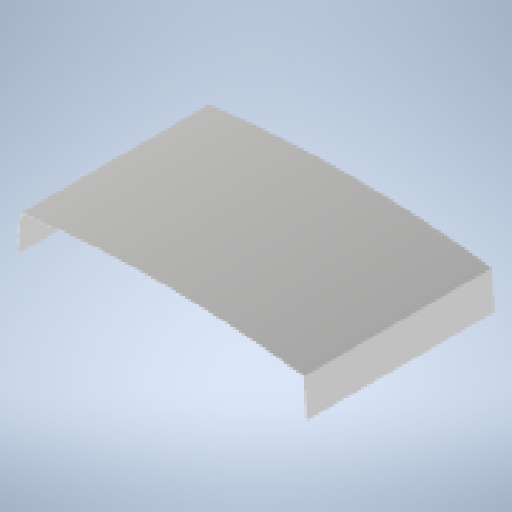
# Autodesk Inventor part: МОО 010 лист спина 1
Saved by Autodesk Inventor 2024.2 (Build 282272000, 272)
## iProperties
Created: 2024-04-18
Part Number: МОО 010 лист спина 1
Material: Stainless Steel AISI 304
Document SubType Name: Sheet Metal
Designer: admin
Density: 8 g/cm^3
Flat Pattern Width: 100 cm
Flat Pattern Length: 190.053 cm
Flat Pattern Area: 19005.3 cm^2
Sheet Metal Rule: Default_mm
Sheet Metal Width: 1000,000 mm
Sheet Metal Length: 1900,535 mm
Sheet Metal Area: 1900534,780 mm^2
Appearance: Default
Mass: 48037.2 g
Surface Area: 40211.1 cm^2
Volume: 6004.65 cm^3
Stock Number: МОО 010 лист спина 1
Author: admin
Autodesk Inventor part; units mm, degrees
ref_plane "YZ Plane" through (0, 0, 0) normal (1, 0, 0) x (0, 1, 0)
ref_plane "XZ Plane" through (0, 0, 0) normal (0, 1, 0) x (-1, 0, 0)
ref_plane "XY Plane" through (0, 0, 0) normal (0, 0, 1) x (1, 0, 0)
sketch "Sketch1" plane through (0, 0, 0) normal (0, 0, 1) x (1, 0, 0)
  line L0 (-800, -50) -> (800, -50) construction
  line L1 (800, -50) -> (800, 0) construction
  line L2 (800, 0) -> (-800, 0) construction
  line L3 (-800, 0) -> (-800, -50) construction
  arc A0 (750, -50) -> (-750, -50) centre (0, -5650) ccw
  arc A1 (-750, -50) -> (-752.5925, -52.7381) centre (-749.6018, -52.9735) ccw
  line L4 (-752.5925, -52.7381) -> (-767.6567, -244.1462)
  arc A2 (752.5925, -52.7381) -> (750, -50) centre (749.6018, -52.9735) ccw
  line L5 (752.5925, -52.7381) -> (767.6567, -244.1462)
  line L6 (0, 0) -> (0, -50) construction
  dimension "d0" = 1600
  dimension "d1" = 50
  dimension "d2" = 50
  dimension "d14" = 3
  dimension "d15" = 192
  dimension "d16" = 94.5
  measures "d0" distance of L2.end L1.end
  measures "d1" distance of L1.end L0.end
  measures "d2" distance of L0.start A0.end
  measures "d14" radius of A1
  measures "d15" distance of L4.start L4.end
  measures "d16" angle of L4 L0
contour flange "Contour Flange1" sketch "Sketch1" thickness 3 bend radius 3 width 1000 along (0, 0, 1) mid plane no both sides no wall seen from (760.1246, -148.4421, 0) lies toward (0.9969173, 0.0784591, 0) curves L5 A2 A0 A1 L4
bend "Bend1"
corner "Corner1"
equation "\"d2\" = d1"
equation "\"d14\" = BendRadius"
equation "\"d3\" = Thickness"
equation "\"d4\" = BendReliefWidth"
equation "\"d5\" = BendReliefDepth"
equation "\"d6\" = MinimumRemnant"
equation "\"d7\" = TransitionRadius"
equation "\"d9\" = BendRadius"
equation "\"d11\" = CornerReliefSize"
equation "\"d12\" = GapSize"
equation "\"d13\" = JacobiRadiusSize"
equation "\"BendRadius\" = Thickness"
equation "\"BendReliefWidth\" = Thickness"
equation "\"BendReliefDepth\" = 0.5 * Thickness"
equation "\"CornerReliefSize\" = 4 * Thickness"
equation "\"MinimumRemnant\" = 2 * Thickness"
equation "\"TransitionRadius\" = BendRadius"
equation "\"JacobiRadiusSize\" = BendRadius"
equation "\"GapSize\" = Thickness"
equation "\"Thickness\" = 3"
body "Solid1"
